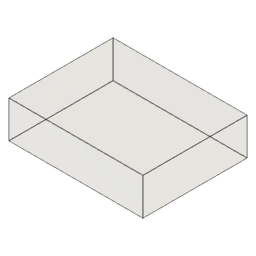
FL CAM Revised version (Autodesk Fusion 360 archive; units mm, degrees)
design "Upright stock 9x7x2.5"
Autodesk Fusion 360 part; units mm, degrees
sketch "Sketch1" plane through (0, 0, 0) normal (0, 0, 1) x (1, 0, 0)
  line L0 (114.3, 88.9) -> (-114.3, 88.9)
  line L1 (-114.3, 88.9) -> (-114.3, -88.9)
  line L2 (-114.3, -88.9) -> (114.3, -88.9)
  line L3 (114.3, -88.9) -> (114.3, 88.9)
  line L4 (114.3, 88.9) -> (-114.3, -88.9) construction
  line L5 (-114.3, 88.9) -> (114.3, -88.9) construction
  dimension "d1" = 228.6
  dimension "d2" = 177.8
  constraint horizontal L0
  constraint perpendicular L0 L1
  constraint parallel L0 L2
  constraint parallel L1 L3
  constraint coincident L4 origin
  constraint coincident L5 origin
  measures "d1" distance of L0.start L0.end
  measures "d2" distance of L0.end L1.end
extrude "Extrude1" add sketch "Sketch1" along normal blind 63.5
